Autodesk Inventor part; units mm, degrees
(part 2 of 2)
sketch "Sketch6" plane through (0, 6.35, 0) normal (0, 0, 1) x (1, 0, 0)
  circle A0 centre (242.0047, 28.5746) radius 4.7625
  circle A1 centre (242.0047, 28.5746) radius 4.7625
  circle A2 centre (89.6047, 28.5746) radius 4.7625
  circle A3 centre (165.8047, 28.5746) radius 4.7625
  circle A4 centre (278.4229, 41.2746) radius 4.7625
  circle A5 centre (278.4229, 15.8746) radius 4.7625
  circle A6 centre (278.4229, 15.8746) radius 4.7625
  circle A7 centre (278.4229, 41.2746) radius 4.7625
  circle A8 centre (406.3903, 28.5746) radius 4.7625
  circle A9 centre (406.3903, 28.5746) radius 4.7625
  circle A10 centre (431.7903, 28.5746) radius 4.7625
  circle A11 centre (431.7903, 28.5746) radius 4.7625
  circle A12 centre (457.1903, 28.5746) radius 4.7625
  circle A13 centre (457.1903, 28.5746) radius 4.7625
  circle A14 centre (572.1571, 28.5746) radius 4.7625
  circle A15 centre (572.1571, 28.5746) radius 4.7625
  circle A16 centre (203.9047, 28.5746) radius 4.7625
  circle A17 centre (203.9047, 28.5746) radius 4.7625
  circle A18 centre (381.8635, 28.5375) radius 3.2004
  circle A19 centre (591.2071, 28.5746) radius 1.016
  circle A20 centre (553.1071, 28.5746) radius 1.016
  circle A21 centre (585.6275, 42.045) radius 1.016
  circle A22 centre (572.1571, 47.6246) radius 1.016
  circle A23 centre (558.6867, 42.045) radius 1.016
  circle A24 centre (484.1537, 12.6996) radius 3.2385
  circle A25 centre (484.1537, 28.5746) radius 3.2385
  circle A26 centre (484.1537, 44.4496) radius 3.2385
  circle A27 centre (506.3546, 28.5746) radius 4.7625
  circle A28 centre (506.3546, 28.5746) radius 4.7625
  circle A29 centre (314.9685, 28.5746) radius 4.7625
  circle A30 centre (314.9685, 28.5746) radius 4.7625
  circle A31 centre (350.0441, 41.2746) radius 4.7625
  circle A32 centre (350.0441, 15.8746) radius 4.7625
  circle A33 centre (350.0441, 15.8746) radius 4.7625
  circle A34 centre (350.0441, 41.2746) radius 4.7625
  circle A35 centre (127.7047, 28.5746) radius 3.2004
  line L0 (673.1, -3.175) -> (0, -3.175)
  line L1 (0, -3.175) -> (0, 60.325)
  line L2 (0, 60.325) -> (673.1, 60.325)
  line L3 (673.1, 60.325) -> (673.1, -3.175)
  line L4 (634.3604, 18.6527) -> (606.6642, 18.6527)
  line L5 (606.6642, 18.6527) -> (606.6642, 38.4965)
  line L6 (606.6642, 38.4965) -> (634.3604, 38.4965)
  line L7 (634.3604, 38.4965) -> (634.3604, 18.6527)
  line L8 (539.6921, 25.2653) -> (528.2621, 25.2653)
  line L9 (528.2621, 25.2653) -> (528.2621, 31.8839)
  line L10 (528.2621, 31.8839) -> (539.6921, 31.8839)
  line L11 (539.6921, 31.8839) -> (539.6921, 25.2653)
  arc A36 (528.2621, 25.2653) -> (539.6921, 25.2653) centre (533.9771, 28.5746) ccw
  arc A37 (539.6921, 31.8839) -> (528.2621, 31.8839) centre (533.9771, 28.5746) ccw
  arc A38 (528.2621, 25.2653) -> (539.6921, 25.2653) centre (533.9771, 28.5746) ccw
  arc A39 (528.2621, 25.2653) -> (539.6921, 25.2653) centre (533.9771, 28.5746) ccw
  circle A40 centre (600.6686, 28.5746) radius 1.651
  line L12 (606.6642, 38.4965) -> (634.3604, 38.4965)
  line L13 (606.6642, 18.6527) -> (634.3604, 18.6527)
  line L14 (634.3604, 38.4965) -> (634.3604, 18.6527)
  circle A41 centre (640.3561, 28.5746) radius 1.651
  line L15 (606.6642, 38.4965) -> (606.6642, 18.6527)
  line L16 (539.6921, 31.8839) -> (539.6921, 25.2653)
  line L17 (528.2621, 31.8839) -> (528.2621, 25.2653)
  arc A42 (528.2621, 31.8839) -> (539.6921, 31.8839) centre (533.9771, 28.5746) cw
  arc A43 (539.6921, 25.2653) -> (528.2621, 25.2653) centre (533.9771, 28.5746) cw
  point P0 (0, -6.35)
  constraints: 40 centre point, 24 end point, 8 point on circle, 4 parallel, 2 concentric, 2 horizontal, 2 perpendicular, 6 other
extrude "Cut2" cut sketch "Sketch6" against normal blind 3.175 contours A0 | A2 | A3 | A4 | A5 | A8 | A10 | A12 | A14 | A16 | A18 | A24 | A25 | A26 | A27 | A29 | A31 | A32 | A35 | L4 L5 L6 L7 | A36 L8 | L8 L9 L10 L11 | L10 A37 | A40 | A41
sketch "Sketch7" plane through (673.1, 6.35, -215.9) normal (0, 0, -1) x (-1, 0, 0)
  circle A0 centre (485.775, 12.573) radius 3.175
  circle A1 centre (485.775, 44.577) radius 3.175
  circle A2 centre (485.775, 28.575) radius 3.175
  circle A3 centre (485.775, 28.575) radius 3.175
  circle A4 centre (485.775, 44.577) radius 3.175
  circle A5 centre (485.775, 12.573) radius 3.175
  circle A6 centre (631.825, 41.275) radius 4.7625
  circle A7 centre (600.075, 28.575) radius 4.7625
  circle A8 centre (561.975, 28.575) radius 4.7625
  circle A9 centre (631.825, 15.875) radius 4.7625
  circle A10 centre (631.825, 15.875) radius 4.7625
  circle A11 centre (561.975, 28.575) radius 4.7625
  circle A12 centre (600.075, 28.575) radius 4.7625
  circle A13 centre (631.825, 41.275) radius 4.7625
  circle A14 centre (523.875, 28.575) radius 4.7625
  circle A15 centre (523.875, 28.575) radius 4.7625
  circle A16 centre (415.925, 28.575) radius 4.7625
  circle A17 centre (301.625, 28.575) radius 4.7625
  circle A18 centre (225.425, 28.575) radius 4.7625
  circle A19 centre (263.525, 28.575) radius 4.7625
  circle A20 centre (339.725, 28.575) radius 4.7625
  circle A21 centre (377.825, 28.575) radius 4.7625
  circle A22 centre (454.025, 28.575) radius 4.7625
  circle A23 centre (454.025, 28.575) radius 4.7625
  circle A24 centre (377.825, 28.575) radius 4.7625
  circle A25 centre (339.725, 28.575) radius 4.7625
  circle A26 centre (263.525, 28.575) radius 4.7625
  circle A27 centre (225.425, 28.575) radius 4.7625
  circle A28 centre (301.625, 28.575) radius 4.7625
  circle A29 centre (415.925, 28.575) radius 4.7625
  circle A30 centre (88.9, 28.575) radius 3.9624
  circle A31 centre (88.9, 28.575) radius 3.9624
  line L0 (673.1, -3.175) -> (0, -3.175)
  line L1 (0, -3.175) -> (0, 60.325)
  line L2 (0, 60.325) -> (673.1, 60.325)
  line L3 (673.1, 60.325) -> (673.1, -3.175)
  circle A32 centre (187.325, 28.575) radius 4.7625
  arc A33 (37.3482, 34.7524) -> (38.8518, 34.7524) centre (38.1, 28.575) ccw
  arc A34 (62.7482, 34.7524) -> (64.2518, 34.7524) centre (63.5, 28.575) ccw
  line L4 (37.3482, 34.7524) -> (37.3482, 33.7364)
  line L5 (38.8518, 33.7364) -> (38.8518, 34.7524)
  line L6 (37.3482, 34.7524) -> (37.3482, 33.7364)
  line L7 (38.8518, 33.7364) -> (38.8518, 34.7524)
  line L8 (37.3482, 34.7524) -> (37.3482, 33.7364)
  line L9 (38.8518, 33.7364) -> (38.8518, 34.7524)
  arc A35 (37.3482, 34.7524) -> (38.8518, 34.7524) centre (38.1, 28.575) ccw
  line L10 (37.3482, 34.7524) -> (37.3482, 33.7364)
  line L11 (38.8518, 33.7364) -> (38.8518, 34.7524)
  line L12 (38.8518, 33.7364) -> (37.3482, 33.7364)
  circle A36 centre (38.1, 28.575) radius 6.223 construction
  line L13 (38.8518, 33.7364) -> (37.3482, 33.7364)
  line L14 (37.3482, 33.7364) -> (37.3482, 34.7524)
  line L15 (37.3482, 34.7524) -> (38.8518, 34.7524)
  line L16 (38.8518, 34.7524) -> (38.8518, 33.7364)
  circle A37 centre (63.5, 28.575) radius 6.223 construction
  line L17 (64.2518, 33.7364) -> (62.7482, 33.7364)
  line L18 (62.7482, 33.7364) -> (62.7482, 34.7524)
  line L19 (62.7482, 34.7524) -> (64.2518, 34.7524)
  line L20 (64.2518, 34.7524) -> (64.2518, 33.7364)
  line L21 (64.2518, 34.7524) -> (62.7482, 34.7524)
  arc A38 (62.7482, 34.7524) -> (64.2518, 34.7524) centre (63.5, 28.575) ccw
  line L22 (62.7482, 33.7364) -> (64.2518, 33.7364)
  arc A39 (62.7482, 34.7524) -> (64.2518, 34.7524) centre (63.5, 28.575) ccw
  line L23 (64.2518, 33.7364) -> (64.2518, 34.7524)
  line L24 (62.7482, 34.7524) -> (62.7482, 33.7364)
  line L25 (37.3482, 33.7364) -> (38.8518, 33.7364)
  arc A40 (37.3482, 34.7524) -> (38.8518, 34.7524) centre (38.1, 28.575) ccw
  line L26 (38.8518, 33.7364) -> (38.8518, 34.7524)
  line L27 (37.3482, 34.7524) -> (37.3482, 33.7364)
  point P0 (673.1, -6.35)
  constraints: 44 end point, 39 centre point, 15 point on circle, 4 parallel, 4 vertical, 3 concentric, 3 horizontal, 3 perpendicular, 2 coincident, 7 other
extrude "Cut3" cut sketch "Sketch7" against normal blind 3.175 contours A0 | A1 | A2 | A6 | A7 | A8 | A9 | A14 | A16 | A17 | A18 | A19 | A20 | A21 | A22 | A30 | A32 | L4 L12 L5 A33 | L18 L17 L20 A34
equation "\"d33\" = Thickness"
equation "\"d35\" = Thickness"
equation "\"d37\" = Thickness"
equation "\"d2\" = Thickness"
equation "\"d3\" = BendReliefWidth"
equation "\"d4\" = BendReliefDepth"
equation "\"d5\" = MinimumRemnant"
equation "\"d6\" = TransitionRadius"
equation "\"d9\" = BendRadius"
equation "\"d10\" = CornerReliefSize"
equation "\"d11\" = GapSize"
equation "\"d12\" = JacobiRadiusSize"
equation "\"d13\" = BendReliefWidth"
equation "\"d14\" = BendReliefDepth"
equation "\"d15\" = MinimumRemnant"
equation "\"d16\" = TransitionRadius"
equation "\"d19\" = BendRadius"
equation "\"d20\" = CornerReliefSize"
equation "\"d21\" = GapSize"
equation "\"d22\" = JacobiRadiusSize"
equation "\"d23\" = BendReliefWidth"
equation "\"d24\" = BendReliefDepth"
equation "\"d25\" = MinimumRemnant"
equation "\"d26\" = TransitionRadius"
equation "\"d29\" = BendRadius"
equation "\"d30\" = CornerReliefSize"
equation "\"d31\" = GapSize"
equation "\"d32\" = JacobiRadiusSize"
equation "\"BendRadius\" = Thickness"
equation "\"BendReliefWidth\" = Thickness"
equation "\"BendReliefDepth\" = 0.5 * Thickness"
equation "\"CornerReliefSize\" = 4 * Thickness"
equation "\"MinimumRemnant\" = 2 * Thickness"
equation "\"TransitionRadius\" = BendRadius"
equation "\"JacobiRadiusSize\" = BendRadius"
equation "\"GapSize\" = Thickness"
equation "\"Thickness\" = 3.175"
body "Solid1"
